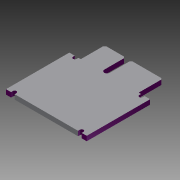
# Autodesk Inventor part: HDMI Plugin Module
Saved by Autodesk Inventor 2015 (Build 190159000, 159)
## iProperties
Created: 2015-10-14
Part Number: HDMI Plugin Module
Material: Generic
Document SubType Name: Modeling
Designer: -
Density: 1 g/cm^3
Appearance: Default
Author: -
Autodesk Inventor part; units mm, degrees
ref_plane "YZ Plane" through (0, 0, 0) normal (1, 0, 0) x (0, 1, 0)
ref_plane "XZ Plane" through (0, 0, 0) normal (0, 1, 0) x (-1, 0, 0)
ref_plane "XY Plane" through (0, 0, 0) normal (0, 0, 1) x (1, 0, 0)
sketch "Sketch1" plane through (0, 0, 0) normal (0, 1, 0) x (-1, 0, 0)
  line L0 (0, 0) -> (-28.321, 0) construction
  line L1 (-28.321, 0) -> (-28.321, -22.225)
  line L2 (-28.321, -22.225) -> (0, -22.225) construction
  line L3 (0, -22.225) -> (0, 0)
  line L4 (-1.778, 0) -> (-3.048, 0) construction
  line L5 (-3.048, 0) -> (-3.048, -0.635)
  line L6 (-2.413, -1.27) -> (-2.413, -1.27)
  line L7 (-1.778, -0.635) -> (-1.778, 0)
  arc A0 (-2.413, -1.27) -> (-1.778, -0.635) centre (-2.413, -0.635) ccw
  arc A1 (-3.048, -0.635) -> (-2.413, -1.27) centre (-2.413, -0.635) ccw
  line L8 (0, 0) -> (-1.778, 0)
  line L9 (0, -11.1125) -> (-6.6148, -11.1125) construction
  line L10 (-14.1605, -22.225) -> (-14.1605, -12.0846) construction
  line L11 (-25.273, 0) -> (-26.543, 0) construction
  line L12 (-26.543, 0) -> (-26.543, -0.635)
  line L13 (-25.908, -1.27) -> (-25.908, -1.27)
  line L14 (-25.273, -0.635) -> (-25.273, 0)
  arc A2 (-25.908, -1.27) -> (-25.273, -0.635) centre (-25.908, -0.635) ccw
  arc A3 (-26.543, -0.635) -> (-25.908, -1.27) centre (-25.908, -0.635) ccw
  line L15 (-26.543, 0) -> (-28.321, 0)
  line L16 (-25.273, 0) -> (-3.048, 0)
  line L17 (-25.146, -22.225) -> (-26.416, -22.225) construction
  line L18 (-26.416, -22.225) -> (-26.416, -21.59)
  line L19 (-25.781, -20.955) -> (-25.781, -20.955)
  line L20 (-25.146, -21.59) -> (-25.146, -22.225)
  line L21 (-1.905, -22.225) -> (-3.175, -22.225) construction
  line L22 (-3.175, -22.225) -> (-3.175, -21.59)
  line L23 (-2.54, -20.955) -> (-2.54, -20.955)
  line L24 (-1.905, -21.59) -> (-1.905, -22.225)
  line L25 (0, -22.225) -> (-1.905, -22.225)
  arc A4 (-1.905, -21.59) -> (-2.54, -20.955) centre (-2.54, -21.59) ccw
  arc A5 (-2.54, -20.955) -> (-3.175, -21.59) centre (-2.54, -21.59) ccw
  arc A6 (-25.146, -21.59) -> (-25.781, -20.955) centre (-25.781, -21.59) ccw
  arc A7 (-25.781, -20.955) -> (-26.416, -21.59) centre (-25.781, -21.59) ccw
  line L26 (-26.416, -22.225) -> (-28.321, -22.225)
  line L27 (-4.0005, -22.225) -> (-24.3205, -22.225) construction
  line L28 (-24.3205, -22.225) -> (-24.3205, -30.099)
  line L29 (-23.8125, -30.607) -> (-4.5085, -30.607) construction
  line L30 (-4.0005, -30.099) -> (-4.0005, -22.225)
  line L31 (-4.5085, -30.607) -> (-4.0005, -30.099)
  line L32 (-23.8125, -30.607) -> (-24.3205, -30.099)
  line L33 (-11.303, -30.607) -> (-13.208, -30.607) construction
  line L34 (-13.208, -30.099) -> (-13.208, -23.1775)
  line L35 (-12.2555, -22.225) -> (-12.2555, -22.225)
  line L36 (-11.303, -23.1775) -> (-11.303, -30.099)
  arc A8 (-12.2555, -22.225) -> (-13.208, -23.1775) centre (-12.2555, -23.1775) ccw
  arc A9 (-11.303, -23.1775) -> (-12.2555, -22.225) centre (-12.2555, -23.1775) ccw
  line L37 (-13.716, -30.607) -> (-23.8125, -30.607)
  line L38 (-10.795, -30.607) -> (-4.5085, -30.607)
  line L39 (-4.0005, -22.225) -> (-3.175, -22.225)
  line L40 (-25.146, -22.225) -> (-24.3205, -22.225)
  line L41 (-10.795, -30.607) -> (-11.303, -30.099)
  line L42 (-13.208, -30.099) -> (-13.716, -30.607)
  point P0 (-2.413, 0)
  point P1 (-26.543, -1.27)
  point P2 (-25.273, -1.27)
  point P3 (-25.908, 0)
  point P4 (-2.54, -22.225)
  point P5 (-25.781, -22.225)
  point P6 (-24.3205, -30.607)
  point P7 (-4.0005, -30.607)
  point P8 (-13.208, -22.225)
  dimension "d0" = 22.225
  dimension "d1" = 28.321
  dimension "d2" = 1.27
  dimension "d3" = 2.413
  dimension "d4" = 1.27
  dimension "d5" = 0.635
  dimension "d6" = 1.27
  dimension "d7" = 1.27
  dimension "d8" = 2.413
  dimension "d9" = 0.635
  dimension "d12" = 1.27
  dimension "d13" = 1.27
  dimension "d14" = 1.27
  dimension "d15" = 1.27
  dimension "d16" = 2.54
  dimension "d17" = 0.635
  dimension "d18" = 2.54
  dimension "d19" = 0.635
  dimension "d20" = 20.32
  dimension "d21" = 0.508
  dimension "d22" = 0.508
  dimension "d23" = 0.508
  dimension "d24" = 0.508
  dimension "d25" = 8.382
  dimension "d26" = 1.905
  dimension "d27" = 0.9525
  dimension "d28" = 8.255
  dimension "d29" = 0.508
  dimension "d30" = 0.508
  dimension "d31" = 0.508
  dimension "d32" = 0.508
  dimension "d40" = 23.495
  constraints: 86 end point, 20 point on circle, 20 tangent, 17 point on line, 14 parallel, 12 collinear, 10 centre point, 10 horizontal, 7 midpoint, 7 perpendicular, 5 concentric, 1 coincident, 1 vertical
  measures "d0" distance of L2.end L0.start
  measures "d1" distance of L0.start L0.end
  measures "d2" distance between parallel lines of L5 L7
  measures "d3" distance of point (-2.413, 0) point (0, 0)
  measures "d4" distance between parallel lines of L0 L6
  measures "d5" radius of A0
  measures "d6" distance of point (-25.273, -1.27) point (-26.543, -1.27)
  measures "d7" distance between parallel lines of L0 L13
  measures "d8" distance of L0.end point (-25.908, 0)
  measures "d9" radius of A2
  measures "d12" distance between parallel lines of L22 L24
  measures "d13" distance between parallel lines of L18 L20
  measures "d14" distance between parallel lines of L17 L19
  measures "d15" distance between parallel lines of L23 L21
  measures "d16" distance of L2.end point (-2.54, -22.225)
  measures "d17" radius of A4
  measures "d18" distance of L1.end point (-25.781, -22.225)
  measures "d19" radius of A6
  measures "d20" distance between parallel lines of L30 L28
  measures "d21" distance of L29.end point (-4.001, -30.607)
  measures "d22" distance of L30.start point (-4.001, -30.607)
  measures "d23" distance of L29.start point (-24.321, -30.607)
  measures "d24" distance of L28.end point (-24.321, -30.607)
  measures "d25" distance between parallel lines of L27 L29
  measures "d26" distance between parallel lines of L34 L36
  measures "d27" radius of A8
  measures "d28" distance from line of L30 A9.centre
  measures "d29" distance of L38.start L33.start
  measures "d30" distance of L36.end L33.start
  measures "d31" distance of L34.start L33.end
  measures "d32" distance of L37.start L33.end
  measures "d40" distance of A2.centre A0.centre
extrude "Extrusion1" add sketch "Sketch1" along normal blind 1.64
sketch "Sketch2" plane through (0, 1.64, 0) normal (0, 1, 0) x (1, 0, 0)
  line L0 (6, -1) -> (22.321, -1)
  line L1 (22.321, -1) -> (22.321, 6)
  line L2 (22.321, 6) -> (6, 6)
  line L3 (6, 6) -> (6, -1)
  line L4 (0, 22.225) -> (0, 0) projected
  line L5 (28.321, 0) -> (28.321, 22.225) projected
  line L6 (3.048, 0) -> (25.273, 0) projected
  dimension "d35" = 7
  dimension "d36" = 6
  dimension "d37" = 6
  dimension "d38" = 1
  constraints: 8 end point, 2 parallel, 1 horizontal, 1 perpendicular
  measures "d35" distance between parallel lines of L0 L2
  measures "d36" distance between parallel lines of L4 L3
  measures "d37" distance between parallel lines of L5 L1
  measures "d38" distance between parallel lines of L6 L0
equation "\"d22\" = d21"
equation "\"d23\" = d21"
equation "\"d24\" = d23"
equation "\"d30\" = d29"
equation "\"d31\" = d29"
equation "\"d32\" = d31"
body "Solid1"
